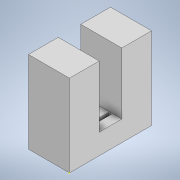
# Autodesk Inventor part: Intsragam
Saved by Autodesk Inventor 2020 (Build 240168000, 168)
## iProperties
Created: 2020-01-07
Part Number: Intsragam
Material: Générique
Document SubType Name: Modeling
Designer: laura
Density: 1 g/cm^3
Appearance: Par défaut
Author: laura
Autodesk Inventor part; units mm, degrees
ref_plane "YZ Plane" through (0, 0, 0) normal (1, 0, 0) x (0, 1, 0)
ref_plane "XZ Plane" through (0, 0, 0) normal (0, 1, 0) x (-1, 0, 0)
ref_plane "XY Plane" through (0, 0, 0) normal (0, 0, 1) x (1, 0, 0)
sketch "Esquisse1" plane through (0, 0, 0) normal (0, 1, 0) x (-1, 0, 0)
  line L0 (0, 0) -> (-40, 0)
  line L1 (-40, 0) -> (-40, -80)
  line L2 (-40, -80) -> (0, -80)
  line L3 (0, -80) -> (0, 0)
  dimension "d0" = 80
  dimension "d4" = 40
  constraints: 8 end point, 2 parallel, 1 horizontal, 1 perpendicular
  measures "d0" distance between parallel lines of L2 L0
  measures "d4" distance between parallel lines of L1 L3
extrude "Extrusion1" add sketch "Esquisse1" along normal blind 80
sketch "Esquisse2" plane through (40, 0, 0) normal (1, 0, 0) x (0, 0, -1)
  point P0 (0, 0)
sketch "Esquisse3" plane through (40, 0, 0) normal (1, 0, 0) x (0, 0, -1)
  line L0 (0, 80) -> (80, 80) projected
  line L1 (20, 20) -> (60, 20)
  line L2 (60, 20) -> (60, 80)
  line L3 (60, 80) -> (20, 80)
  line L4 (20, 80) -> (20, 20)
  line L5 (0, 0) -> (80, 0) projected
  line L6 (80, 0) -> (80, 80) projected
  line L7 (0, 0) -> (0, 80) projected
  point P0 (20, 80)
  dimension "d9" = 20
  dimension "d10" = 20
  dimension "d11" = 20
  constraints: 8 end point, 2 parallel, 1 horizontal, 1 perpendicular, 1 point on line
  measures "d9" distance between parallel lines of L5 L1
  measures "d10" distance between parallel lines of L6 L2
  measures "d11" distance between parallel lines of L7 L4
extrude "Extrusion2" cut sketch "Esquisse3" against normal blind 80 contours L0 L2 L1 L4
sketch "Esquisse4" plane through (40, 20, -20) normal (0, 1, 0) x (1, 0, 0)
  line L0 (0, 40) -> (-40, 40) projected
  line L1 (0, 0) -> (-5, 0)
  line L2 (-5, 40) -> (0, 40)
  line L3 (0, 40) -> (0, 0)
  line L4 (-5, 40) -> (-10, 40)
  line L5 (-9, 10) -> (-12, 10)
  line L6 (-12, 10) -> (-12, 30)
  line L7 (-12, 30) -> (-9, 30)
  line L8 (-9, 10) -> (-9, 30)
  point P0 (-40, -20)
  dimension "d19" = 20
  dimension "d21" = 9
  dimension "d22" = 3
  constraints: 16 end point, 2 horizontal, 2 vertical, 1 parallel, 1 point on line
  measures "d19" distance of L5.end L6.end
  measures "d21" distance between parallel lines of L8 L3
  measures "d22" distance of L5.start L5.end
extrude "Extrusion3" cut sketch "Esquisse4" against normal blind 10
sketch "Esquisse6" plane through (40, 20, -20) normal (0, 0, -1) x (-1, 0, 0)
  line L0 (40, 60) -> (40, 0) projected
  line L1 (0, 60) -> (40, 60) projected
  line L2 (0, 0) -> (0, 60) projected
  line L3 (0, 0) -> (40, 0) projected
  point P0 (40, -20)
extrude "Extrusion4" add sketch "Esquisse6" along normal blind 9
sketch "Esquisse7" plane through (40, 20, -60) normal (0, 0, 1) x (1, 0, 0)
  line L0 (-40, 0) -> (-40, 60) projected
  line L1 (0, 0) -> (-40, 0) projected
  line L2 (0, 60) -> (0, 0) projected
  line L3 (-40, 60) -> (0, 60) projected
  point P0 (-40, -20)
extrude "Extrusion5" add sketch "Esquisse7" along normal blind 9
